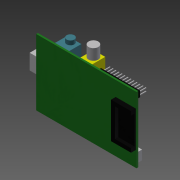
# Autodesk Inventor part: Raspi
Saved by Autodesk Inventor 2016 (Build 200138000, 138)
## iProperties
Created: 2014-02-08
Part Number: Raspi
Material: Steel, Mild
Document SubType Name: Modeling
Designer: Jack
Density: 7.86 g/cm^3
Appearance: Steel
Author: Jack
Autodesk Inventor part; units mm, degrees
ref_plane "YZ Plane" through (0, 0, 0) normal (1, 0, 0) x (0, 1, 0)
ref_plane "XZ Plane" through (0, 0, 0) normal (0, 1, 0) x (-1, 0, 0)
ref_plane "XY Plane" through (0, 0, 0) normal (0, 0, 1) x (1, 0, 0)
sketch "Sketch1" plane through (0, 0, 0) normal (0, 1, 0) x (-1, 0, 0)
  line L0 (0, 0) -> (85, 0)
  line L1 (85, 0) -> (85, 56)
  line L2 (85, 56) -> (0, 56)
  line L3 (0, 56) -> (0, 0)
  dimension "d0" = 85
  dimension "d1" = 56
  constraints: 8 end point, 2 parallel, 1 horizontal, 1 perpendicular
  measures "d0" distance of L0.start L0.end
  measures "d1" distance of L0.end L1.end
extrude "Extrusion1" add sketch "Sketch1" along normal blind 1.5
sketch "Sketch2" plane through (0, 1.5, 0) normal (0, 1, 0) x (1, 0, 0)
  line L0 (0, 0) -> (-85, 0) projected
  line L1 (-85, 0) -> (-85, -56) projected
  line L2 (-86, -2) -> (-65, -2)
  line L3 (-65, -2) -> (-65, -18)
  line L4 (-65, -18) -> (-86, -18)
  line L5 (-86, -18) -> (-86, -2)
  dimension "d4" = 21
  dimension "d5" = 16
  dimension "d6" = 1
  dimension "d7" = 2
  constraints: 8 end point, 2 parallel, 1 horizontal, 1 perpendicular
  measures "d4" distance of L2.start L2.end
  measures "d5" distance of L2.end L3.end
  measures "d6" distance between parallel lines of L1 L5
  measures "d7" distance between parallel lines of L0 L2
extrude "Extrusion2" add sketch "Sketch2" along normal blind 13.5
sketch "Sketch3" plane through (0, 1.5, 0) normal (0, 1, 0) x (1, 0, 0)
  line L0 (-85, -18) -> (-85, -56) projected
  line L1 (-85, -56) -> (0, -56) projected
  line L2 (-92, -25) -> (-75, -25)
  line L3 (-75, -25) -> (-75, -38)
  line L4 (-75, -38) -> (-92, -38)
  line L5 (-92, -38) -> (-92, -25)
  dimension "d10" = 17
  dimension "d11" = 13
  dimension "d12" = 7
  dimension "d13" = 18
  constraints: 8 end point, 2 parallel, 1 horizontal, 1 perpendicular
  measures "d10" distance of L2.start L2.end
  measures "d11" distance of L2.end L3.end
  measures "d12" distance between parallel lines of L0 L5
  measures "d13" distance between parallel lines of L1 L4
extrude "Extrusion3" add sketch "Sketch3" along normal blind 15.5
sketch "Sketch4" plane through (0, 1.5, 0) normal (0, 1, 0) x (1, 0, 0)
  line L0 (-85, -38) -> (-85, -56) projected
  line L1 (-85, -56) -> (0, -56) projected
  line L2 (-70.5, -44.5) -> (-58.5, -44.5)
  line L3 (-58.5, -44.5) -> (-58.5, -56)
  line L4 (-58.5, -56) -> (-70.5, -56)
  line L5 (-70.5, -56) -> (-70.5, -44.5)
  dimension "d16" = 11.5
  dimension "d17" = 12
  dimension "d18" = 14.5
  constraints: 8 end point, 2 parallel, 1 collinear, 1 horizontal, 1 perpendicular
  measures "d16" distance of L4.end L2.start
  measures "d17" distance of L2.start L2.end
  measures "d18" distance between parallel lines of L0 L5
extrude "Extrusion4" add sketch "Sketch4" along normal blind 10.3
sketch "Sketch5" plane through (-85, 0, 56) normal (0, 0, 1) x (1, 0, 0)
  line L0 (14.5, 11.8) -> (26.5, 11.8) projected
  line L1 (14.5, 1.5) -> (14.5, 11.8) projected
  line L2 (0, 0) -> (0, 1.5) projected
  line L3 (14.5, 1.5) -> (26.5, 1.5)
  circle A0 centre (20.5, 8.55) radius 3.25
  dimension "d21" = 6.5
  dimension "d23" = 6
  constraints: 2 end point, 1 centre point, 1 perpendicular, 1 tangent
  measures "d21" diameter of A0
  measures "d23" distance from line of L1 A0.centre
extrude "Extrusion5" add sketch "Sketch5" along normal blind 3.5
sketch "Sketch6" plane through (0, 1.5, 0) normal (0, 1, 0) x (1, 0, 0)
  line L0 (-58.5, -56) -> (0, -56) projected
  line L1 (-85, -38) -> (-85, -56) projected
  line L2 (-51, -44) -> (-41, -44)
  line L3 (-41, -44) -> (-41, -54)
  line L4 (-41, -54) -> (-51, -54)
  line L5 (-51, -54) -> (-51, -44)
  dimension "d26" = 10
  dimension "d27" = 10
  dimension "d28" = 34
  dimension "d29" = 2
  constraints: 8 end point, 2 parallel, 1 horizontal, 1 perpendicular
  measures "d26" distance of L2.start L2.end
  measures "d27" distance of L4.end L2.start
  measures "d28" distance between parallel lines of L1 L5
  measures "d29" distance between parallel lines of L0 L4
extrude "Extrusion6" add sketch "Sketch6" along normal blind 13
sketch "Sketch7" plane through (-85, 0, 56) normal (0, 0, 1) x (1, 0, 0)
  line L0 (26.5, 1.5) -> (26.5, 11.8) projected
  line L1 (20.5, 11.8) -> (26.5, 11.8) projected
  circle A0 centre (20.5, 8.55) radius 3.25 projected
  line L2 (14.5, 11.8) -> (20.5, 11.8) projected
  line L3 (14.5, 1.5) -> (14.5, 11.8) projected
  line L4 (0, 0) -> (0, 1.5) projected
  line L5 (14.5, 1.5) -> (26.5, 1.5)
  constraints: 2 end point, 1 perpendicular, 1 vertical alignment
extrude "Extrusion7" cut sketch "Sketch7" against normal blind 0.01
sketch "Sketch8" plane through (-51, 1.5, 54) normal (0, 0, 1) x (1, 0, 0)
  line L0 (0, 13) -> (10, 13) projected
  circle A0 centre (5, 8) radius 4.125
  point P0 (51, -1.5)
  dimension "d34" = 8.25
  dimension "d35" = 5
  constraints: 1 centre point
  measures "d34" diameter of A0
  measures "d35" distance from line of L0 A0.centre
extrude "Extrusion8" add sketch "Sketch8" along normal blind 9.25
sketch "Sketch9" plane through (0, 1.5, 0) normal (0, 1, 0) x (1, 0, 0)
  line L0 (-85, -56) -> (0, -56) projected
  line L1 (0, -56) -> (0, 0) projected
  line L2 (-34, -54.5) -> (-1, -54.5)
  line L3 (-1, -54.5) -> (-1, -49.6)
  line L4 (-1, -49.6) -> (-34, -49.6)
  line L5 (-34, -49.6) -> (-34, -54.5)
  dimension "d38" = 4.9
  dimension "d39" = 33
  dimension "d40" = 1.5
  dimension "d41" = 1
  constraints: 8 end point, 2 parallel, 1 horizontal, 1 perpendicular
  measures "d38" distance of L2.end L3.end
  measures "d39" distance of L3.end L4.end
  measures "d40" distance between parallel lines of L0 L2
  measures "d41" distance between parallel lines of L1 L3
extrude "Extrusion9" add sketch "Sketch9" along normal blind 2.5
sketch "Sketch10" plane through (0, 4, 0) normal (0, 1, 0) x (1, 0, 0)
  line L0 (-1, -54.5) -> (-1, -49.6) projected
  line L1 (-1, -49.6) -> (-34, -49.6) projected
  line L2 (-34, -49.6) -> (-34, -54.5) projected
  line L3 (-2.2, -50.2) -> (-1.6, -50.2)
  line L4 (-1.6, -50.2) -> (-1.6, -50.8)
  line L5 (-1.6, -50.8) -> (-2.2, -50.8)
  line L6 (-2.2, -50.8) -> (-2.2, -50.2)
  line L7 (-4.7385, -50.2) -> (-4.1385, -50.2)
  line L8 (-4.1385, -50.2) -> (-4.1385, -50.8)
  line L9 (-4.1385, -50.8) -> (-4.7385, -50.8)
  line L10 (-4.7385, -50.8) -> (-4.7385, -50.2)
  line L11 (-7.2769, -50.2) -> (-6.6769, -50.2)
  line L12 (-6.6769, -50.2) -> (-6.6769, -50.8)
  line L13 (-6.6769, -50.8) -> (-7.2769, -50.8)
  line L14 (-7.2769, -50.8) -> (-7.2769, -50.2)
  line L15 (-9.8154, -50.2) -> (-9.2154, -50.2)
  line L16 (-9.2154, -50.2) -> (-9.2154, -50.8)
  line L17 (-9.2154, -50.8) -> (-9.8154, -50.8)
  line L18 (-9.8154, -50.8) -> (-9.8154, -50.2)
  line L19 (-12.3538, -50.2) -> (-11.7538, -50.2)
  line L20 (-11.7538, -50.2) -> (-11.7538, -50.8)
  line L21 (-11.7538, -50.8) -> (-12.3538, -50.8)
  line L22 (-12.3538, -50.8) -> (-12.3538, -50.2)
  line L23 (-14.8923, -50.2) -> (-14.2923, -50.2)
  line L24 (-14.2923, -50.2) -> (-14.2923, -50.8)
  line L25 (-14.2923, -50.8) -> (-14.8923, -50.8)
  line L26 (-14.8923, -50.8) -> (-14.8923, -50.2)
  line L27 (-17.4308, -50.2) -> (-16.8308, -50.2)
  line L28 (-16.8308, -50.2) -> (-16.8308, -50.8)
  line L29 (-16.8308, -50.8) -> (-17.4308, -50.8)
  line L30 (-17.4308, -50.8) -> (-17.4308, -50.2)
  line L31 (-19.9692, -50.2) -> (-19.3692, -50.2)
  line L32 (-19.3692, -50.2) -> (-19.3692, -50.8)
  line L33 (-19.3692, -50.8) -> (-19.9692, -50.8)
  line L34 (-19.9692, -50.8) -> (-19.9692, -50.2)
  line L35 (-22.5077, -50.2) -> (-21.9077, -50.2)
  line L36 (-21.9077, -50.2) -> (-21.9077, -50.8)
  line L37 (-21.9077, -50.8) -> (-22.5077, -50.8)
  line L38 (-22.5077, -50.8) -> (-22.5077, -50.2)
  line L39 (-25.0461, -50.2) -> (-24.4461, -50.2)
  line L40 (-24.4461, -50.2) -> (-24.4461, -50.8)
  line L41 (-24.4461, -50.8) -> (-25.0461, -50.8)
  line L42 (-25.0461, -50.8) -> (-25.0461, -50.2)
  line L43 (-27.5846, -50.2) -> (-26.9846, -50.2)
  line L44 (-26.9846, -50.2) -> (-26.9846, -50.8)
  line L45 (-26.9846, -50.8) -> (-27.5846, -50.8)
  line L46 (-27.5846, -50.8) -> (-27.5846, -50.2)
  line L47 (-30.1231, -50.2) -> (-29.5231, -50.2)
  line L48 (-29.5231, -50.2) -> (-29.5231, -50.8)
  line L49 (-29.5231, -50.8) -> (-30.1231, -50.8)
  line L50 (-30.1231, -50.8) -> (-30.1231, -50.2)
  line L51 (-32.6615, -50.2) -> (-32.0615, -50.2)
  line L52 (-32.0615, -50.2) -> (-32.0615, -50.8)
  line L53 (-32.0615, -50.8) -> (-32.6615, -50.8)
  line L54 (-32.6615, -50.8) -> (-32.6615, -50.2)
  line L55 (-2.2, -52.8) -> (-1.6, -52.8)
  line L56 (-1.6, -52.8) -> (-1.6, -53.4)
  line L57 (-1.6, -53.4) -> (-2.2, -53.4)
  line L58 (-2.2, -53.4) -> (-2.2, -52.8)
  line L59 (-4.7385, -52.8) -> (-4.1385, -52.8)
  line L60 (-4.1385, -52.8) -> (-4.1385, -53.4)
  line L61 (-4.1385, -53.4) -> (-4.7385, -53.4)
  line L62 (-4.7385, -53.4) -> (-4.7385, -52.8)
  line L63 (-7.2769, -52.8) -> (-6.6769, -52.8)
  line L64 (-6.6769, -52.8) -> (-6.6769, -53.4)
  line L65 (-6.6769, -53.4) -> (-7.2769, -53.4)
  line L66 (-7.2769, -53.4) -> (-7.2769, -52.8)
  line L67 (-9.8154, -52.8) -> (-9.2154, -52.8)
  line L68 (-9.2154, -52.8) -> (-9.2154, -53.4)
  line L69 (-9.2154, -53.4) -> (-9.8154, -53.4)
  line L70 (-9.8154, -53.4) -> (-9.8154, -52.8)
  line L71 (-12.3538, -52.8) -> (-11.7538, -52.8)
  line L72 (-11.7538, -52.8) -> (-11.7538, -53.4)
  line L73 (-11.7538, -53.4) -> (-12.3538, -53.4)
  line L74 (-12.3538, -53.4) -> (-12.3538, -52.8)
  line L75 (-14.8923, -52.8) -> (-14.2923, -52.8)
  line L76 (-14.2923, -52.8) -> (-14.2923, -53.4)
  line L77 (-14.2923, -53.4) -> (-14.8923, -53.4)
  line L78 (-14.8923, -53.4) -> (-14.8923, -52.8)
  line L79 (-17.4308, -52.8) -> (-16.8308, -52.8)
  line L80 (-16.8308, -52.8) -> (-16.8308, -53.4)
  line L81 (-16.8308, -53.4) -> (-17.4308, -53.4)
  line L82 (-17.4308, -53.4) -> (-17.4308, -52.8)
  line L83 (-19.9692, -52.8) -> (-19.3692, -52.8)
  line L84 (-19.3692, -52.8) -> (-19.3692, -53.4)
  line L85 (-19.3692, -53.4) -> (-19.9692, -53.4)
  line L86 (-19.9692, -53.4) -> (-19.9692, -52.8)
  line L87 (-22.5077, -52.8) -> (-21.9077, -52.8)
  line L88 (-21.9077, -52.8) -> (-21.9077, -53.4)
  line L89 (-21.9077, -53.4) -> (-22.5077, -53.4)
  line L90 (-22.5077, -53.4) -> (-22.5077, -52.8)
  line L91 (-25.0461, -52.8) -> (-24.4461, -52.8)
  line L92 (-24.4461, -52.8) -> (-24.4461, -53.4)
  line L93 (-24.4461, -53.4) -> (-25.0461, -53.4)
  line L94 (-25.0461, -53.4) -> (-25.0461, -52.8)
  line L95 (-27.5846, -52.8) -> (-26.9846, -52.8)
  line L96 (-26.9846, -52.8) -> (-26.9846, -53.4)
  line L97 (-26.9846, -53.4) -> (-27.5846, -53.4)
  line L98 (-27.5846, -53.4) -> (-27.5846, -52.8)
  line L99 (-30.1231, -52.8) -> (-29.5231, -52.8)
  line L100 (-29.5231, -52.8) -> (-29.5231, -53.4)
  line L101 (-29.5231, -53.4) -> (-30.1231, -53.4)
  line L102 (-30.1231, -53.4) -> (-30.1231, -52.8)
  line L103 (-32.6615, -52.8) -> (-32.0615, -52.8)
  line L104 (-32.0615, -52.8) -> (-32.0615, -53.4)
  line L105 (-32.0615, -53.4) -> (-32.6615, -53.4)
  line L106 (-32.6615, -53.4) -> (-32.6615, -52.8)
  point P0 (0, 0)
  dimension "d44" = 0.6
  dimension "d45" = 0.6
  dimension "d46" = 0.6
  dimension "d47" = 0.6
  dimension "d50" = 2.5385
  dimension "d53" = 2.6
  constraints: 208 end point, 2 horizontal, 2 parallel, 1 perpendicular, 1 vertical, 200 other
  measures "d44" distance of L3.start L3.end
  measures "d45" distance of L5.end L3.start
  measures "d46" distance between parallel lines of L0 L4
  measures "d47" distance between parallel lines of L1 L3
  measures "d50" distance of L3.start L7.start
  measures "d53" distance of L3.start L55.start
extrude "Extrusion10" add sketch "Sketch10" along normal blind 6
sketch "Sketch11" plane through (0, 0, 0) normal (0, -1, 0) x (1, 0, 0)
  line L0 (0, 56) -> (0, 0) projected
  line L1 (-85, 56) -> (0, 56) projected
  line L2 (-0.6, 13.1) -> (-17.6, 13.1)
  line L3 (-17.6, 13.1) -> (-17.6, 43.5)
  line L4 (-17.6, 43.5) -> (-0.6, 43.5)
  line L5 (-0.6, 43.5) -> (-0.6, 13.1)
  dimension "d58" = 30.4
  dimension "d59" = 17
  dimension "d60" = 0.6
  dimension "d61" = 12.5
  constraints: 8 end point, 2 parallel, 1 horizontal, 1 perpendicular
  measures "d58" distance of L2.end L3.end
  measures "d59" distance of L3.end L4.end
  measures "d60" distance between parallel lines of L0 L5
  measures "d61" distance between parallel lines of L1 L4
extrude "Extrusion11" add sketch "Sketch11" along normal blind 4
sketch "Sketch12" plane through (0, -4, 0) normal (0, -1, 0) x (1, 0, 0)
  line L0 (-0.6, 13.1) -> (-0.6, 43.5) projected
  line L1 (-0.6, 43.5) -> (-17.6, 43.5) projected
  line L2 (-17.6, 43.5) -> (-17.6, 13.1) projected
  line L3 (-0.6, 40.3) -> (-14.3, 40.3)
  line L4 (-14.3, 40.3) -> (-14.3, 16.3)
  line L5 (-14.3, 16.3) -> (-0.6, 16.3)
  point P0 (0, 0)
  dimension "d64" = 13.7
  dimension "d65" = 24
  dimension "d66" = 3.2
  constraints: 6 end point, 3 perpendicular, 2 point on line
  measures "d64" distance of L3.start L3.end
  measures "d65" distance of L3.end L4.end
  measures "d66" distance between parallel lines of L3 L1
extrude "Extrusion12" cut sketch "Sketch12" against normal blind 2.9
sketch "Sketch13" plane through (0, 1.5, 0) normal (0, 1, 0) x (1, 0, 0)
  line L0 (0, -56) -> (0, 0) projected
  line L1 (0, 0) -> (-85, 0) projected
  line L2 (-5.4, -3.6) -> (0.2, -3.6)
  line L3 (0.2, -3.6) -> (0.2, -11.6)
  line L4 (0.2, -11.6) -> (-5.4, -11.6)
  line L5 (-5.4, -11.6) -> (-5.4, -3.6)
  dimension "d69" = 5.6
  dimension "d70" = 8
  dimension "d71" = 3.6
  dimension "d72" = 0.2
  constraints: 8 end point, 2 parallel, 1 horizontal, 1 perpendicular
  measures "d69" distance of L2.start L2.end
  measures "d70" distance of L2.end L3.end
  measures "d71" distance between parallel lines of L1 L2
  measures "d72" distance between parallel lines of L0 L3
extrude "Extrusion13" add sketch "Sketch13" along normal blind 3
sketch "Sketch14" plane through (0, 1.5, 0) normal (0, 1, 0) x (1, 0, 0)
  line L0 (0, 0) -> (-85, 0) projected
  line L1 (-85, 0) -> (-85, -2) projected
  line L2 (-51, 0.8) -> (-36, 0.8)
  line L3 (-36, 0.8) -> (-36, -10.7)
  line L4 (-36, -10.7) -> (-51, -10.7)
  line L5 (-51, -10.7) -> (-51, 0.8)
  dimension "d75" = 15
  dimension "d76" = 11.5
  dimension "d77" = 0.8
  dimension "d78" = 34
  constraints: 8 end point, 2 parallel, 1 horizontal, 1 perpendicular
  measures "d75" distance of L2.start L2.end
  measures "d76" distance of L2.end L3.end
  measures "d77" distance between parallel lines of L0 L2
  measures "d78" distance between parallel lines of L1 L5
extrude "Extrusion14" add sketch "Sketch14" along normal blind 6
sketch "Sketch15" plane through (0, 1.5, 0) normal (0, 1, 0) x (1, 0, 0)
  line L0 (-51, 0) -> (-85, 0) projected
  line L1 (-85, 0) -> (-85, -2) projected
  line L2 (-59, 0) -> (-55, 0)
  line L3 (-55, 0) -> (-55, -22)
  line L4 (-55, -22) -> (-59, -22)
  line L5 (-59, -22) -> (-59, 0)
  dimension "d81" = 22
  dimension "d82" = 4
  dimension "d83" = 26
  constraints: 8 end point, 2 parallel, 1 collinear, 1 horizontal, 1 perpendicular
  measures "d81" distance of L4.end L2.start
  measures "d82" distance of L2.start L2.end
  measures "d83" distance between parallel lines of L1 L5
extrude "Extrusion15" add sketch "Sketch15" along normal blind 7
sketch "Sketch16" plane through (0, 0, 0) normal (0, 0, -1) x (-1, 0, 0)
  line L0 (59, 1.5) -> (59, 8.5) projected
  line L1 (55, 8.5) -> (59, 8.5) projected
  line L2 (55, 1.5) -> (55, 8.5) projected
  line L3 (0, 0) -> (0, 1.5) projected
  line L4 (55, 1.5) -> (59, 1.5)
  constraints: 2 end point, 1 perpendicular
extrude "Extrusion16" cut sketch "Sketch16" against normal blind 0.01
body "Solid1"
